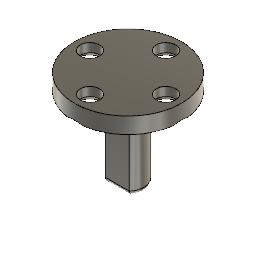
ServoHornAdapter (Autodesk Fusion 360 design; units mm, degrees)
Autodesk Fusion 360 part; units mm, degrees
sketch "Sketch1" plane through (0, 0, 0) normal (0, 0, 1) x (1, 0, 0)
  circle A0 centre (0, 0) radius 10
  dimension "d1" = 20
  constraint coincident A0.centre origin
  measures "d1" diameter of A0
extrude "Extrude1" add sketch "Sketch1" along normal blind 3
sketch "Sketch2" plane through (0, 0, 0) normal (0, 0, -1) x (1, 0, 0)
  circle A0 centre (0, 0) radius 10
  line L0 (-2.2361, 2) -> (2.2361, 2)
  line L1 (2.2361, -2) -> (-2.2361, -2)
  arc A1 (-2.2361, 2) -> (-2.2361, -2) centre (0, 0) ccw
  arc A2 (2.2361, -2) -> (2.2361, 2) centre (0, 0) ccw
  dimension "d4" = 6
  dimension "d5" = 4
  constraint concentric A0 A1
  constraint horizontal L0
  constraint coincident L1.start A1
  constraint parallel L0 L1
  constraint equal L0 L1
  constraint concentric A1 A2
  measures "d4" diameter of A1
  measures "d5" distance of L0 L1
extrude "Extrude2" add sketch "Sketch2" along normal blind 15 contours L0 L1 A1 A2
fillet "Fillet1" radius 1 4 edges at (0, -2, 0) (3, 0, 0) (-3, 0, 0) (0, 2, 0)
fillet "Fillet1" radius 0.9 4 edges at (0, -2, -15) (3, 0, -15) (0, 2, -15) (-3, 0, -15)
sketch "Sketch3" plane through (0, 0, 0) normal (0, 0, -1) x (1, 0, 0)
  circle A0 centre (0, 0) radius 10
  line L0 (-2.6458, 3) -> (2.6458, 3)
  arc A1 (2.6458, -3) -> (2.6458, 3) centre (0, 0) ccw
  line L1 (2.6458, -3) -> (-2.6458, -3)
  arc A2 (-2.6458, 3) -> (-2.6458, -3) centre (0, 0) ccw
  point P0 (-7.1, 0)
  dimension "d10" = 7.1
  measures "d10" distance of A0.centre P0
hole "Hole1" at (-7.1, 0, 0) direction (0, 0, 1) diameter 3.6 depth 12 tip angle 118 countersink diameter 6.3 countersink angle 90
pattern_circular "C-Pattern1" count 4 over 360 about axis through (0, 0, 1.75) along (0, 0, 1) of "Hole1"
